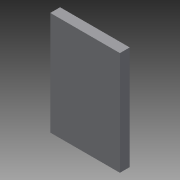
# Autodesk Inventor part: ankerpro15000mah
Saved by Autodesk Inventor 2015 (Build 190159000, 159)
## iProperties
Created: 2014-09-17
Part Number: ankerpro15000mah
Material: Generic
Document SubType Name: Modeling
Designer: ericd_000
Density: 1 g/cm^3
Appearance: Default
Author: ericd_000
Autodesk Inventor part; units mm, degrees
ref_plane "YZ Plane" through (0, 0, 0) normal (1, 0, 0) x (0, 1, 0)
ref_plane "XZ Plane" through (0, 0, 0) normal (0, 1, 0) x (-1, 0, 0)
ref_plane "XY Plane" through (0, 0, 0) normal (0, 0, 1) x (1, 0, 0)
sketch "Sketch1" plane through (0, 0, 0) normal (0, 1, 0) x (-1, 0, 0)
  line L0 (45.6548, 67.5635) -> (-53.4452, 67.5635)
  line L1 (-53.4452, 67.5635) -> (-53.4452, -79.9365)
  line L2 (-53.4452, -79.9365) -> (45.6548, -79.9365)
  line L3 (45.6548, -79.9365) -> (45.6548, 67.5635)
  point P0 (0, 0)
  dimension "d0" = 147.5
  dimension "d1" = 99.1
  constraints: 8 end point, 2 parallel, 1 horizontal, 1 perpendicular
  measures "d0" distance of L2.end L0.start
  measures "d1" distance of L0.start L0.end
extrude "Extrusion1" add sketch "Sketch1" along normal blind 14
body "Solid1"
